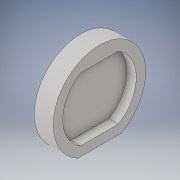
# Autodesk Inventor part: end cap
Saved by Autodesk Inventor 2017 (Build 210142000, 142)
## iProperties
Created: 2018-03-04
Part Number: end cap
Material: Generic
Document SubType Name: Modeling
Designer: Braxton
Density: 1 g/cm^3
Appearance: Default
Author: Braxton
Autodesk Inventor part; units mm, degrees
ref_plane "YZ Plane" through (0, 0, 0) normal (1, 0, 0) x (0, 1, 0)
ref_plane "XZ Plane" through (0, 0, 0) normal (0, 1, 0) x (-1, 0, 0)
ref_plane "XY Plane" through (0, 0, 0) normal (0, 0, 1) x (1, 0, 0)
sketch "Sketch1" plane through (0, 0, 0) normal (1, 0, 0) x (0, 1, 0)
  line L0 (-84.6667, -50.8) -> (-84.6667, 50.8)
  line L1 (84.6667, -50.8) -> (84.6667, 50.8)
  arc A0 (-110.0667, -57.4059) -> (-110.0667, 57.4059) centre (0, 0) ccw
  arc A1 (-84.6667, -50.8) -> (84.6667, -50.8) centre (0, 0) ccw
  arc A2 (84.6667, 50.8) -> (-84.6667, 50.8) centre (0, 0) ccw
  line L2 (-110.0667, 57.4059) -> (-110.0667, -57.4059)
  dimension "d12" = 169.3333
  dimension "d13" = 101.6
  dimension "d18" = 25.4
  constraints: 6 end point, 6 point on circle, 3 centre point, 2 coincident, 1 parallel, 1 vertical
  measures "d12" distance between parallel lines of L1 L0
  measures "d13" distance of L0.start L0.end
  measures "d18" distance between parallel lines of L0 L2
extrude "Extrusion4" add sketch "Sketch1" along normal blind 25.4
sketch "Sketch5" plane through (0, 0, 0) normal (-1, 0, 0) x (0, 0, -1)
  arc A0 (-57.4059, 110.0667) -> (57.4059, 110.0667) centre (0, 0) ccw
  line L0 (-57.4059, 110.0667) -> (57.4059, 110.0667) projected
  line L1 (-57.4059, 110.0667) -> (57.4059, 110.0667)
  constraints: 2 end point, 2 point on circle, 1 centre point, 1 coincident, 1 collinear
extrude "Extrusion5" add sketch "Sketch5" along normal blind 25.4
body "Solid2"
